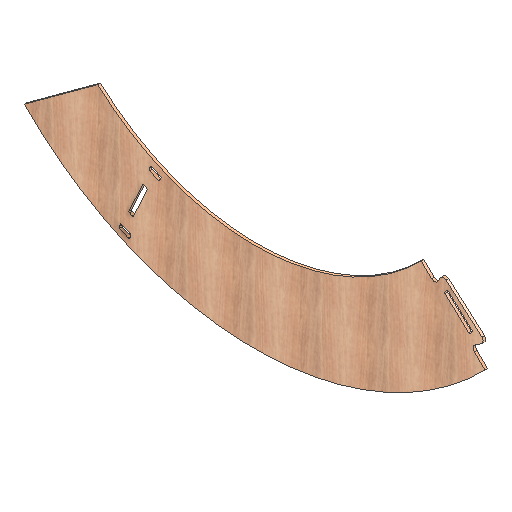
# Autodesk Inventor part: Platform C1
Saved by Autodesk Inventor 2021 (Build 250183000, 183)
## iProperties
Created: 2020-05-09
Part Number: Platform C1
Material: Wood (Birch)
Document SubType Name: Modeling
Designer: Dan Wikman
Density: 0.55 g/cm^3
Appearance: Birch - Natural Polished
Mass: 3085.21 g
Surface Area: 11708.7 cm^2
Volume: 5609.47 cm^3
Autodesk Inventor part; units mm, degrees
ref_plane "YZ Plane" through (0, 0, 0) normal (1, 0, 0) x (0, 1, 0)
ref_plane "XZ Plane" through (0, 0, 0) normal (0, 1, 0) x (-1, 0, 0)
ref_plane "XY Plane" through (0, 0, 0) normal (0, 0, 1) x (1, 0, 0)
sketch "CONTOURS" plane through (0, 0, 0) normal (0, 0, 1) x (1, 0, 0)
  line L0 (1957.6292, 879.0874) -> (1973.7702, 879.0874)
  arc A0 (1973.7702, 871.0874) -> (1973.7702, 879.0874) centre (1973.7702, 875.0874) ccw
  line L1 (2395.2631, 344.4855) -> (2395.2631, 361.2856)
  line L2 (2395.2631, 361.2856) -> (2335.4041, 361.2856)
  arc A1 (2327.4041, 361.2857) -> (2335.4041, 361.2856) centre (2331.4041, 361.2856) ccw
  line L3 (2327.4041, 361.2857) -> (2327.4041, 413.0854)
  arc A2 (2046.6196, 767.5507) -> (2327.4041, 413.0854) centre (2780.5524, 1060.4825) ccw
  arc A3 (2046.6196, 767.5507) -> (2038.9046, 766.0679) centre (2042.9046, 766.0679) ccw
  line L4 (2038.9046, 766.0679) -> (2038.9041, 604.8116)
  line L5 (2038.9041, 604.8116) -> (2060.9041, 604.8116)
  arc A4 (2068.9041, 604.8116) -> (2060.9041, 604.8116) centre (2064.9041, 604.8116) ccw
  line L6 (2068.9041, 604.8116) -> (2068.9041, 585.8116)
  arc A5 (2060.9041, 585.8116) -> (2068.9041, 585.8116) centre (2064.9041, 585.8116) ccw
  line L7 (2060.9041, 585.8116) -> (2037.4041, 585.8116)
  line L8 (2037.4041, 585.8116) -> (1996.4234, 585.8116)
  arc A6 (1988.9234, 587.8213) -> (1996.4234, 585.8116) centre (1996.4234, 600.8116) ccw
  line L9 (1988.9234, 587.8213) -> (1963.7631, 602.3475)
  arc A7 (1963.7631, 602.3475) -> (1957.7631, 598.8834) centre (1961.7631, 598.8834) ccw
  line L10 (1957.7631, 598.8834) -> (1957.7631, 403.7398)
  arc A8 (1957.7631, 403.7398) -> (1963.7631, 400.2757) centre (1961.7631, 403.7398) ccw
  line L11 (1963.7631, 400.2757) -> (1988.9234, 414.802)
  arc A9 (1996.4234, 416.8116) -> (1988.9234, 414.802) centre (1996.4234, 401.8116) ccw
  line L12 (1996.4234, 416.8116) -> (2037.4041, 416.8116)
  line L13 (2037.4041, 416.8116) -> (2060.9041, 416.8116)
  arc A10 (2068.9041, 416.8116) -> (2060.9041, 416.8116) centre (2064.9041, 416.8116) ccw
  line L14 (2068.9041, 416.8116) -> (2068.9041, 397.8116)
  arc A11 (2060.9041, 397.8116) -> (2068.9041, 397.8116) centre (2064.9041, 397.8116) ccw
  line L15 (2060.9041, 397.8116) -> (2038.9041, 397.8116)
  line L16 (2038.9041, 397.8116) -> (2038.9041, 210.8117)
  line L17 (2038.9041, 210.8117) -> (2052.4041, 210.8117)
  arc A12 (2052.4041, 202.8117) -> (2052.4041, 210.8117) centre (2052.4041, 206.8117) ccw
  line L18 (2052.4041, 202.8117) -> (2052.4041, 195.3488)
  arc A13 (2052.4041, 195.3488) -> (2327.4041, 47.9742) centre (2799.5688, 1259.2914) ccw
  arc A14 (2327.4041, 39.9742) -> (2327.4041, 47.9742) centre (2327.4041, 43.9742) ccw
  line L19 (2327.4041, 39.9742) -> (2327.4041, 23.2856)
  line L20 (2327.4041, 23.2856) -> (2395.2631, 23.2856)
  line L21 (2395.2631, 23.2856) -> (2395.2631, 40.0855)
  arc A15 (2395.2631, 48.0855) -> (2395.2631, 40.0855) centre (2395.2631, 44.0855) ccw
  line L22 (2395.2631, 48.0855) -> (2411.4041, 48.0855)
  line L23 (2411.4041, 48.0855) -> (2411.4041, 66.0855)
  line L24 (2411.4041, 66.0855) -> (2403.2631, 66.0855)
  arc A16 (2395.2631, 66.0855) -> (2403.2631, 66.0855) centre (2399.2631, 66.0855) ccw
  line L25 (2395.2631, 66.0855) -> (2395.2631, 132.0783)
  line L26 (2395.2631, 132.0783) -> (2373.2631, 132.0783)
  arc A17 (2365.2631, 132.0783) -> (2373.2631, 132.0783) centre (2369.2631, 132.0783) ccw
  line L27 (2365.2631, 132.0783) -> (2365.2631, 148.6501)
  line L28 (2365.2631, 148.6501) -> (2364.8394, 148.4335)
  line L29 (2364.8394, 148.4335) -> (2364.4234, 148.2026)
  line L30 (2364.4234, 148.2026) -> (2339.2631, 133.6763)
  arc A18 (2331.7631, 138.0065) -> (2339.2631, 133.6763) centre (2336.7631, 138.0065) ccw
  line L31 (2331.7631, 138.0065) -> (2331.7631, 246.5646)
  arc A19 (2339.2631, 250.8947) -> (2331.7631, 246.5646) centre (2336.7631, 246.5646) ccw
  line L32 (2339.2631, 250.8947) -> (2364.4234, 236.3684)
  line L33 (2364.4234, 236.3684) -> (2364.8394, 236.1375)
  line L34 (2364.8394, 236.1375) -> (2365.2631, 235.9209)
  line L35 (2365.2631, 235.9209) -> (2365.2631, 252.4928)
  arc A20 (2373.2631, 252.4928) -> (2365.2631, 252.4928) centre (2369.2631, 252.4928) ccw
  line L36 (2373.2631, 252.4928) -> (2395.2631, 252.4928)
  line L37 (2395.2631, 252.4928) -> (2395.2631, 318.4855)
  arc A21 (2403.2631, 318.4855) -> (2395.2631, 318.4855) centre (2399.2631, 318.4855) ccw
  line L38 (2403.2631, 318.4855) -> (2411.4041, 318.4855)
  line L39 (2411.4041, 318.4855) -> (2411.4041, 336.4855)
  line L40 (2411.4041, 336.4855) -> (2395.2631, 336.4855)
  arc A22 (2395.2631, 344.4855) -> (2395.2631, 336.4855) centre (2395.2631, 340.4855) ccw
  line L41 (1973.7702, 871.0874) -> (1973.7702, 854.2874)
  line L42 (1973.7702, 854.2874) -> (2033.6292, 854.2873)
  line L43 (2041.6292, 854.2873) -> (2041.6292, 802.4876)
  arc A23 (2322.4137, 448.0223) -> (2041.6292, 802.4876) centre (1588.4809, 155.0905) ccw
  arc A24 (2322.4137, 448.0223) -> (2330.1287, 449.505) centre (2326.1287, 449.505) ccw
  line L44 (2330.1287, 449.505) -> (2330.1292, 610.7613)
  line L45 (2330.1292, 610.7613) -> (2308.1292, 610.7613)
  arc A25 (2300.1292, 610.7613) -> (2308.1292, 610.7613) centre (2304.1292, 610.7613) ccw
  line L46 (2300.1292, 610.7613) -> (2300.1292, 629.7613)
  arc A26 (2308.1292, 629.7613) -> (2300.1292, 629.7613) centre (2304.1292, 629.7613) ccw
  line L47 (2308.1292, 629.7613) -> (2331.6292, 629.7613)
  line L48 (2331.6292, 629.7613) -> (2372.6099, 629.7613)
  arc A27 (2380.1099, 627.7517) -> (2372.6099, 629.7613) centre (2372.6099, 614.7613) ccw
  line L49 (2380.1099, 627.7517) -> (2405.2702, 613.2254)
  arc A28 (2405.2702, 613.2254) -> (2411.2702, 616.6895) centre (2407.2702, 616.6895) ccw
  line L50 (2411.2702, 616.6895) -> (2411.2702, 811.8331)
  line L51 (2405.2702, 815.2972) -> (2380.1099, 800.7709)
  arc A29 (2372.6099, 798.7613) -> (2380.1099, 800.7709) centre (2372.6099, 813.7613) ccw
  line L52 (2372.6099, 798.7613) -> (2331.6292, 798.7613)
  line L53 (2331.6292, 798.7613) -> (2308.1292, 798.7613)
  arc A30 (2300.1292, 798.7613) -> (2308.1292, 798.7613) centre (2304.1292, 798.7613) ccw
  line L54 (2300.1292, 798.7613) -> (2300.1292, 817.7613)
  arc A31 (2308.1292, 817.7613) -> (2300.1292, 817.7613) centre (2304.1292, 817.7613) ccw
  line L55 (2308.1292, 817.7613) -> (2330.1292, 817.7613)
  line L56 (2330.1292, 817.7613) -> (2330.1292, 1004.7612)
  line L57 (2330.1292, 1004.7612) -> (2316.6292, 1004.7612)
  arc A32 (2316.6292, 1012.7612) -> (2316.6292, 1004.7612) centre (2316.6292, 1008.7612) ccw
  line L58 (2316.6292, 1012.7612) -> (2316.6292, 1020.2242)
  arc A33 (2316.6292, 1020.2242) -> (2041.6292, 1167.5988) centre (1569.4645, -43.7184) ccw
  arc A34 (2041.6292, 1175.5988) -> (2041.6292, 1167.5988) centre (2041.6292, 1171.5988) ccw
  line L59 (2041.6292, 1175.5988) -> (2041.6292, 1192.2873)
  line L60 (2041.6292, 1192.2873) -> (1973.7702, 1192.2873)
  line L61 (1973.7702, 1192.2873) -> (1973.7702, 1175.4874)
  arc A35 (1973.7702, 1167.4874) -> (1973.7702, 1175.4874) centre (1973.7702, 1171.4874) ccw
  line L62 (1973.7702, 1167.4874) -> (1957.6292, 1167.4874)
  line L63 (1957.6292, 1167.4874) -> (1957.6292, 1149.4874)
  line L64 (1957.6292, 1149.4874) -> (1965.7702, 1149.4874)
  arc A36 (1973.7702, 1149.4874) -> (1965.7702, 1149.4874) centre (1969.7702, 1149.4874) ccw
  line L65 (1973.7702, 1149.4874) -> (1973.7702, 1083.4947)
  line L66 (1973.7702, 1083.4947) -> (1995.7702, 1083.4947)
  arc A37 (2003.7702, 1083.4946) -> (1995.7702, 1083.4947) centre (1999.7702, 1083.4947) ccw
  line L67 (2003.7702, 1083.4946) -> (2003.7702, 1066.9228)
  line L68 (2003.7702, 1066.9228) -> (2004.1939, 1067.1394)
  line L69 (2004.1939, 1067.1394) -> (2004.6099, 1067.3703)
  line L70 (2004.6099, 1067.3703) -> (2029.7702, 1081.8966)
  arc A38 (2037.2702, 1077.5665) -> (2029.7702, 1081.8966) centre (2032.2702, 1077.5665) ccw
  line L71 (2037.2702, 1077.5665) -> (2037.2702, 969.0084)
  line L72 (2029.7702, 964.6782) -> (2004.6099, 979.2045)
  line L73 (2004.6099, 979.2045) -> (2004.1939, 979.4354)
  line L74 (2004.1939, 979.4354) -> (2003.7702, 979.652)
  line L75 (2003.7702, 979.652) -> (2003.7702, 963.0802)
  arc A39 (1995.7702, 963.0802) -> (2003.7702, 963.0802) centre (1999.7702, 963.0802) ccw
  arc A40 (2411.2702, 811.8331) -> (2405.2702, 815.2972) centre (2407.2702, 811.8331) ccw
  line L76 (29.0412, 889.8609) -> (69.6135, 929.6413)
  arc A41 (92.1865, 926.768) -> (69.6135, 929.6413) centre (79.765, 919.2877) ccw
  line L77 (92.1865, 926.768) -> (107.0781, 902.0398)
  arc A42 (107.0781, 902.0398) -> (131.8211, 899.605) centre (120.3563, 910.0361) ccw
  line L78 (131.8211, 899.605) -> (252.9238, 1032.7101)
  arc A43 (252.9238, 1032.7101) -> (248.9601, 1056.7052) centre (241.459, 1043.1412) ccw
  line L79 (248.9601, 1056.7052) -> (234.1791, 1064.8793)
  arc A44 (231.0447, 1087.9218) -> (234.1791, 1064.8793) centre (241.1963, 1077.5683) ccw
  line L80 (231.0447, 1087.9218) -> (270.3869, 1126.4961)
  arc A45 (270.3869, 1126.4961) -> (1527.2637, 1126.4961) centre (898.8253, 1743.5906) ccw
  line L81 (1527.2637, 1126.4961) -> (1815.1018, 939.9773)
  arc A46 (29.0412, 889.8609) -> (1815.1018, 939.9773) centre (898.8169, 1743.6721) ccw
  line L82 (1523.2972, 649.9931) -> (1562.6322, 611.4115)
  arc A47 (1562.6322, 611.4115) -> (1587.1937, 615.2422) centre (1573.4858, 622.4771) ccw
  line L83 (1587.1937, 615.2422) -> (1595.0777, 630.18)
  arc A48 (1617.4481, 634.3255) -> (1595.0777, 630.18) centre (1607.9012, 623.4119) ccw
  line L84 (1617.4481, 634.3255) -> (1752.8919, 515.8444)
  arc A49 (1751.0665, 492.6576) -> (1752.8919, 515.8444) centre (1743.3451, 504.9307) ccw
  line L85 (1751.0665, 492.6576) -> (1726.6337, 477.2861)
  arc A50 (1726.6337, 477.2861) -> (1724.034, 453.1009) centre (1734.8877, 464.1665) ccw
  line L86 (1724.034, 453.1009) -> (1764.599, 413.3129)
  arc A51 (25.3482, 413.3129) -> (1764.599, 413.3129) centre (894.9736, 1267.2896) ccw
  line L87 (25.3482, 413.3129) -> (302.205, 615.759)
  arc A52 (302.205, 615.759) -> (1523.2972, 649.9931) centre (894.9664, 1267.2343) ccw
  line L88 (1995.7702, 963.0802) -> (1973.7702, 963.0802)
  line L89 (1973.7702, 963.0802) -> (1973.7702, 897.0874)
  arc A53 (1965.7702, 897.0874) -> (1973.7702, 897.0874) centre (1969.7702, 897.0874) ccw
  line L90 (1965.7702, 897.0874) -> (1957.6292, 897.0874)
  line L91 (1957.6292, 897.0874) -> (1957.6292, 879.0874)
  dimension "d1" = 338
  dimension "d3" = 16.6885
  dimension "d5" = 18
  dimension "d7" = 16.141
  dimension "d9" = 51.7997
  dimension "d11" = 1300.088
  dimension "d13" = 16.7999
  constraints: 184 end point, 108 point on circle, 54 centre point
  measures "d1" distance of L43.start L59.end
  measures "d3" distance of L59.start L59.end
  measures "d5" distance of L90.end L0.start
  measures "d7" distance from line of L89 L90.end
  measures "d9" distance of L43.start L43.end
  measures "d11" radius of A33
  measures "d13" distance of L60.end L61.end
sketch "HOLES" plane through (0, 0, 0) normal (0, 0, 1) x (1, 0, 0)
  line L0 (417.6052, 171.9081) -> (384.9317, 187.0224)
  arc A0 (382.9807, 192.3322) -> (384.9317, 187.0224) centre (386.6111, 190.6528) ccw
  line L1 (382.9807, 192.3322) -> (387.5989, 202.3157)
  arc A1 (392.9087, 204.2668) -> (387.5989, 202.3157) centre (391.2293, 200.6364) ccw
  line L2 (392.9087, 204.2668) -> (425.5822, 189.1525)
  arc A2 (427.5332, 183.8427) -> (425.5822, 189.1525) centre (423.9028, 185.5221) ccw
  line L3 (290.0252, 1067.7256) -> (282.3828, 1059.8139)
  arc A3 (276.7268, 1059.716) -> (282.3828, 1059.8139) centre (279.5059, 1062.593) ccw
  line L4 (276.7268, 1059.716) -> (250.8342, 1084.7274)
  arc A4 (250.7363, 1090.3834) -> (250.8342, 1084.7274) centre (253.6132, 1087.6044) ccw
  line L5 (250.7363, 1090.3834) -> (258.3786, 1098.2951)
  arc A5 (264.0347, 1098.393) -> (258.3786, 1098.2951) centre (261.2556, 1095.516) ccw
  line L6 (264.0347, 1098.393) -> (289.9273, 1073.3816)
  arc A6 (290.0252, 1067.7256) -> (289.9273, 1073.3816) centre (287.1482, 1070.5046) ccw
  line L7 (102.1615, 873.2431) -> (94.5191, 865.3315)
  arc A7 (88.8631, 865.2335) -> (94.5191, 865.3315) centre (91.6422, 868.1105) ccw
  line L8 (88.8631, 865.2335) -> (62.9705, 890.245)
  arc A8 (62.8726, 895.901) -> (62.9705, 890.245) centre (65.7496, 893.1219) ccw
  line L9 (62.8726, 895.901) -> (70.515, 903.8126)
  arc A9 (76.171, 903.9105) -> (70.515, 903.8126) centre (73.3919, 901.0336) ccw
  line L10 (488.8536, 364.5631) -> (437.7587, 253.7781)
  arc A10 (102.1615, 873.2431) -> (102.0636, 878.8991) centre (99.2846, 876.0221) ccw
  line L11 (1358.4331, 945.869) -> (1353.2703, 955.5821)
  arc A11 (1353.2703, 955.5821) -> (1347.8609, 957.2368) centre (1349.7382, 953.7047) ccw
  line L12 (1347.8609, 957.2368) -> (1316.0723, 940.3404)
  arc A12 (1316.0723, 940.3404) -> (1314.4176, 934.931) centre (1317.9497, 936.8084) ccw
  line L13 (1314.4176, 934.931) -> (1319.5804, 925.2178)
  arc A13 (1319.5804, 925.2178) -> (1324.9899, 923.5631) centre (1323.1125, 927.0952) ccw
  line L14 (1324.9899, 923.5631) -> (1356.7784, 940.4595)
  arc A14 (1356.7784, 940.4595) -> (1358.4331, 945.869) centre (1354.901, 943.9916) ccw
  line L15 (1441.3284, 696.1636) -> (1446.4912, 686.4505)
  arc A15 (1446.4912, 686.4505) -> (1451.9006, 684.7958) centre (1450.0232, 688.3278) ccw
  line L16 (1451.9006, 684.7958) -> (1483.6892, 701.6922)
  arc A16 (1483.6892, 701.6922) -> (1485.3438, 707.1016) centre (1481.8118, 705.2242) ccw
  line L17 (1485.3438, 707.1016) -> (1480.181, 716.8148)
  arc A17 (1480.181, 716.8148) -> (1474.7716, 718.4695) centre (1476.649, 714.9374) ccw
  line L18 (1474.7716, 718.4695) -> (1442.9831, 701.5731)
  arc A18 (1442.9831, 701.5731) -> (1441.3284, 696.1636) centre (1444.8604, 698.041) ccw
  line L19 (1363.2554, 875.1779) -> (1357.078, 871.8854)
  arc A19 (1357.078, 871.8854) -> (1355.4295, 866.4741) centre (1358.9594, 868.3555) ccw
  line L20 (1355.4295, 866.4741) -> (1412.8118, 758.8114)
  arc A20 (1412.8118, 758.8114) -> (1418.2231, 757.1628) centre (1416.3417, 760.6927) ccw
  line L21 (1418.2231, 757.1628) -> (1427.9304, 762.3366)
  arc A21 (1427.9304, 762.3366) -> (1429.579, 767.7479) centre (1426.049, 765.8666) ccw
  line L22 (1429.579, 767.7479) -> (1372.1967, 875.4107)
  arc A22 (1372.1967, 875.4107) -> (1366.7853, 877.0592) centre (1368.6667, 873.5293) ccw
  line L23 (1366.7853, 877.0592) -> (1363.2554, 875.1779)
  line L24 (1703.0768, 505.0739) -> (1613.5973, 588.0042)
  arc A23 (1613.3826, 593.657) -> (1613.5973, 588.0042) centre (1616.3164, 590.938) ccw
  line L25 (1613.3826, 593.657) -> (1620.8599, 601.7248)
  arc A24 (1626.5127, 601.9395) -> (1620.8599, 601.7248) centre (1623.7937, 599.0058) ccw
  line L26 (1626.5127, 601.9395) -> (1715.9922, 519.0093)
  arc A25 (1716.2069, 513.3565) -> (1715.9922, 519.0093) centre (1713.2731, 516.0755) ccw
  line L27 (1716.2069, 513.3565) -> (1708.7296, 505.2887)
  arc A26 (1703.0768, 505.0739) -> (1708.7296, 505.2887) centre (1705.7958, 508.0077) ccw
  line L28 (541.1297, 429.4206) -> (541.1463, 429.4626)
  arc A27 (541.1463, 429.4626) -> (539.1072, 434.5669) centre (537.4278, 430.9365) ccw
  line L29 (539.1072, 434.5669) -> (506.4339, 449.6811)
  arc A28 (506.4339, 449.6811) -> (501.1241, 447.7301) centre (504.7545, 446.0507) ccw
  line L30 (501.1241, 447.7301) -> (496.5059, 437.7465)
  arc A29 (496.5059, 437.7465) -> (498.4569, 432.4368) centre (500.1363, 436.0672) ccw
  line L31 (498.4569, 432.4368) -> (531.1304, 417.3225)
  arc A30 (531.1304, 417.3225) -> (536.4402, 419.2735) centre (532.8098, 420.9529) ccw
  line L32 (536.4402, 419.2735) -> (541.0584, 429.2571)
  line L33 (541.0584, 429.2571) -> (541.0948, 429.338)
  line L34 (541.0948, 429.338) -> (541.1297, 429.4206)
  line L35 (480.54, 372.8023) -> (486.8965, 369.8706)
  arc A31 (488.8536, 364.5631) -> (486.8965, 369.8706) centre (485.2213, 366.2383) ccw
  arc A32 (432.4511, 251.8211) -> (437.7587, 253.7781) centre (434.1264, 255.4533) ccw
  line L36 (432.4511, 251.8211) -> (422.4623, 256.428)
  arc A33 (420.5053, 261.7355) -> (422.4623, 256.428) centre (424.1376, 260.0603) ccw
  line L37 (420.5053, 261.7355) -> (471.6002, 372.5205)
  arc A34 (476.9077, 374.4775) -> (471.6002, 372.5205) centre (475.2325, 370.8452) ccw
  line L38 (476.9077, 374.4775) -> (480.54, 372.8023)
  line L39 (427.5332, 183.8427) -> (422.915, 173.8591)
  arc A35 (417.6052, 171.9081) -> (422.915, 173.8591) centre (419.2846, 175.5385) ccw
  line L40 (76.171, 903.9105) -> (102.0636, 878.8991)
  constraints: 82 end point, 72 point on circle, 36 centre point
sketch "LETTERS" plane through (0, 0, 0) normal (0, 0, 1) x (1, 0, 0)
  line L0 (565.2488, 269.5965) -> (565.4715, 269.5068)
  line L1 (565.4715, 269.5068) -> (565.6923, 269.4126)
  line L2 (565.6923, 269.4126) -> (565.9113, 269.314)
  line L3 (565.9113, 269.314) -> (566.1283, 269.2109)
  line L4 (566.1283, 269.2109) -> (566.3432, 269.1036)
  line L5 (566.3432, 269.1036) -> (566.556, 268.9919)
  line L6 (566.556, 268.9919) -> (566.7665, 268.876)
  line L7 (566.7665, 268.876) -> (566.9747, 268.7559)
  line L8 (566.9747, 268.7559) -> (567.1804, 268.6317)
  line L9 (567.1804, 268.6317) -> (567.3837, 268.5035)
  line L10 (567.3837, 268.5035) -> (567.5843, 268.3713)
  line L11 (567.5843, 268.3713) -> (567.7822, 268.2351)
  line L12 (567.7822, 268.2351) -> (567.9773, 268.095)
  line L13 (567.9773, 268.095) -> (568.1695, 267.951)
  line L14 (568.1695, 267.951) -> (568.3587, 267.8033)
  line L15 (568.3587, 267.8033) -> (568.5449, 267.6519)
  line L16 (568.5449, 267.6519) -> (568.7279, 267.4968)
  line L17 (568.7279, 267.4968) -> (568.9076, 267.3381)
  line L18 (568.9076, 267.3381) -> (569.084, 267.1758)
  line L19 (569.084, 267.1758) -> (569.2569, 267.01)
  line L20 (569.2569, 267.01) -> (569.4263, 266.8407)
  line L21 (569.4263, 266.8407) -> (569.5921, 266.6681)
  line L22 (569.5921, 266.6681) -> (569.7542, 266.4921)
  line L23 (569.7542, 266.4921) -> (569.9124, 266.3129)
  line L24 (569.9124, 266.3129) -> (570.0668, 266.1304)
  line L25 (570.0668, 266.1304) -> (570.2171, 265.9448)
  line L26 (570.2171, 265.9448) -> (570.3634, 265.756)
  line L27 (570.3634, 265.756) -> (570.5054, 265.5642)
  line L28 (570.5054, 265.5642) -> (570.6432, 265.3693)
  line L29 (570.6432, 265.3693) -> (570.7767, 265.1716)
  line L30 (570.7767, 265.1716) -> (570.9058, 264.9711)
  line L31 (570.9058, 264.9711) -> (571.0303, 264.7679)
  line L32 (571.0303, 264.7679) -> (571.1503, 264.5622)
  line L33 (571.1503, 264.5622) -> (571.2656, 264.354)
  line L34 (571.2656, 264.354) -> (571.3762, 264.1435)
  line L35 (571.3762, 264.1435) -> (571.482, 263.9307)
  line L36 (571.482, 263.9307) -> (571.583, 263.7158)
  line L37 (571.583, 263.7158) -> (571.679, 263.4989)
  line L38 (571.679, 263.4989) -> (571.77, 263.28)
  line L39 (571.77, 263.28) -> (571.8558, 263.0594)
  line L40 (571.8558, 263.0594) -> (571.9365, 262.8371)
  line L41 (571.9365, 262.8371) -> (572.012, 262.6132)
  line L42 (572.012, 262.6132) -> (572.0821, 262.3878)
  line L43 (572.0821, 262.3878) -> (572.1469, 262.1611)
  line L44 (572.1469, 262.1611) -> (572.2061, 261.9332)
  line L45 (572.2061, 261.9332) -> (572.2599, 261.7041)
  line L46 (572.2599, 261.7041) -> (572.308, 261.474)
  line L47 (572.308, 261.474) -> (572.3504, 261.2429)
  line L48 (572.3504, 261.2429) -> (572.3871, 261.0111)
  line L49 (572.3871, 261.0111) -> (572.4179, 260.7785)
  line L50 (572.4179, 260.7785) -> (572.4428, 260.5454)
  line L51 (572.4428, 260.5454) -> (572.4617, 260.3118)
  line L52 (572.4617, 260.3118) -> (572.4745, 260.0778)
  line L53 (572.4745, 260.0778) -> (572.4811, 259.8435)
  line L54 (572.4811, 259.8435) -> (572.4816, 259.6092)
  line L55 (572.4816, 259.6092) -> (572.4757, 259.3747)
  line L56 (572.4757, 259.3747) -> (572.4635, 259.1404)
  line L57 (572.4635, 259.1404) -> (572.4449, 258.9062)
  line L58 (572.4449, 258.9062) -> (572.4197, 258.6723)
  line L59 (572.4197, 258.6723) -> (572.3879, 258.4388)
  line L60 (572.3879, 258.4388) -> (572.3494, 258.2058)
  line L61 (572.3494, 258.2058) -> (572.3044, 257.9735)
  line L62 (572.3044, 257.9735) -> (572.2529, 257.7421)
  line L63 (572.2529, 257.7421) -> (572.195, 257.5116)
  line L64 (572.195, 257.5116) -> (572.1308, 257.2824)
  line L65 (572.1308, 257.2824) -> (572.0604, 257.0546)
  line L66 (572.0604, 257.0546) -> (571.9839, 256.8283)
  line L67 (571.9839, 256.8283) -> (571.9014, 256.6037)
  line L68 (571.9014, 256.6037) -> (571.8129, 256.381)
  line L69 (571.8129, 256.381) -> (571.7186, 256.1604)
  line L70 (571.7186, 256.1604) -> (571.6186, 255.9421)
  line L71 (571.6186, 255.9421) -> (571.5129, 255.7261)
  line L72 (571.5129, 255.7261) -> (571.4016, 255.5127)
  line L73 (571.4016, 255.5127) -> (571.2849, 255.3021)
  line L74 (571.2849, 255.3021) -> (571.1628, 255.0944)
  line L75 (571.1628, 255.0944) -> (571.0354, 254.8898)
  line L76 (571.0354, 254.8898) -> (570.9028, 254.6885)
  line L77 (570.9028, 254.6885) -> (570.7652, 254.4906)
  line L78 (570.7652, 254.4906) -> (570.6225, 254.2964)
  line L79 (570.6225, 254.2964) -> (570.4749, 254.106)
  line L80 (570.4749, 254.106) -> (570.3225, 253.9195)
  line L81 (570.3225, 253.9195) -> (570.1654, 253.7372)
  line L82 (570.1654, 253.7372) -> (570.0037, 253.5591)
  line L83 (570.0037, 253.5591) -> (569.8374, 253.3856)
  line L84 (569.8374, 253.3856) -> (569.6667, 253.2167)
  line L85 (569.6667, 253.2167) -> (569.4916, 253.0527)
  line L86 (569.4916, 253.0527) -> (569.3123, 252.8937)
  line L87 (569.3123, 252.8937) -> (569.1288, 252.7398)
  line L88 (569.1288, 252.7398) -> (568.9412, 252.5913)
  line L89 (568.9412, 252.5913) -> (568.7497, 252.4483)
  line L90 (568.7497, 252.4483) -> (568.5543, 252.311)
  line L91 (568.5543, 252.311) -> (568.355, 252.1796)
  line L92 (568.355, 252.1796) -> (568.1521, 252.0542)
  line L93 (568.1521, 252.0542) -> (567.9457, 251.9349)
  line L94 (567.9457, 251.9349) -> (567.736, 251.8219)
  line L95 (567.736, 251.8219) -> (567.5231, 251.715)
  line L96 (567.5231, 251.715) -> (567.3073, 251.6145)
  line L97 (567.3073, 251.6145) -> (567.0888, 251.5204)
  line L98 (567.0888, 251.5204) -> (566.8677, 251.4327)
  line L99 (566.8677, 251.4327) -> (566.6443, 251.3516)
  line L100 (566.6443, 251.3516) -> (566.4187, 251.2771)
  line L101 (566.4187, 251.2771) -> (566.1911, 251.2092)
  line L102 (566.1911, 251.2092) -> (565.9618, 251.1481)
  line L103 (565.9618, 251.1481) -> (565.7308, 251.0938)
  line L104 (565.7308, 251.0938) -> (565.4985, 251.0464)
  line L105 (565.4985, 251.0464) -> (565.265, 251.0059)
  line L106 (565.265, 251.0059) -> (565.0305, 250.9724)
  line L107 (565.0305, 250.9724) -> (564.7951, 250.946)
  line L108 (564.7951, 250.946) -> (564.5591, 250.9268)
  line L109 (564.5591, 250.9268) -> (564.3227, 250.9148)
  line L110 (564.3227, 250.9148) -> (564.0861, 250.9101)
  line L111 (564.0861, 250.9101) -> (563.8494, 250.9127)
  line L112 (563.8494, 250.9127) -> (563.6128, 250.9228)
  line L113 (563.6128, 250.9228) -> (563.3766, 250.9404)
  line L114 (563.1409, 250.9656) -> (562.906, 250.9983)
  line L115 (562.906, 250.9983) -> (562.6719, 251.0388)
  line L116 (562.6719, 251.0388) -> (562.439, 251.0871)
  line L117 (562.439, 251.0871) -> (562.2074, 251.1432)
  line L118 (562.2074, 251.1432) -> (561.9772, 251.2072)
  line L119 (561.9772, 251.2072) -> (561.7487, 251.2792)
  line L120 (561.7487, 251.2792) -> (561.5221, 251.3592)
  line L121 (561.5221, 251.3592) -> (561.2975, 251.4473)
  line L122 (561.2975, 251.4473) -> (561.1861, 251.4945)
  line L123 (561.1861, 251.4945) -> (561.0753, 251.5437)
  line L124 (554.4697, 256.2412) -> (554.3188, 256.4266)
  line L125 (554.3188, 256.4266) -> (554.1731, 256.616)
  line L126 (554.1731, 256.616) -> (554.0329, 256.8093)
  line L127 (554.0329, 256.8093) -> (553.898, 257.0063)
  line L128 (553.898, 257.0063) -> (553.7686, 257.2069)
  line L129 (553.7686, 257.2069) -> (553.6447, 257.411)
  line L130 (553.6447, 257.411) -> (553.5265, 257.6182)
  line L131 (553.5265, 257.6182) -> (553.414, 257.8286)
  line L132 (553.414, 257.8286) -> (553.3071, 258.0418)
  line L133 (553.3071, 258.0418) -> (553.2061, 258.2578)
  line L134 (553.2061, 258.2578) -> (553.1109, 258.4764)
  line L135 (553.1109, 258.4764) -> (553.0217, 258.6974)
  line L136 (553.0217, 258.6974) -> (552.9385, 258.9206)
  line L137 (552.9385, 258.9206) -> (552.8613, 259.1459)
  line L138 (552.8613, 259.1459) -> (552.7902, 259.3732)
  line L139 (563.3766, 250.9404) -> (563.1409, 250.9656)
  line L140 (552.7902, 259.3732) -> (552.7253, 259.6021)
  line L141 (552.7253, 259.6021) -> (552.6667, 259.8327)
  line L142 (552.6667, 259.8327) -> (552.6143, 260.0646)
  line L143 (552.6143, 260.0646) -> (552.5684, 260.2978)
  line L144 (552.5684, 260.2978) -> (552.5289, 260.5321)
  line L145 (552.5289, 260.5321) -> (552.4959, 260.7673)
  line L146 (552.4959, 260.7673) -> (552.4694, 261.0032)
  line L147 (552.4694, 261.0032) -> (552.4496, 261.2397)
  line L148 (552.4496, 261.2397) -> (552.4365, 261.4766)
  line L149 (552.4365, 261.4766) -> (552.4301, 261.7138)
  line L150 (552.4301, 261.7138) -> (552.4305, 261.9511)
  line L151 (552.4305, 261.9511) -> (552.4379, 262.1882)
  line L152 (552.4379, 262.1882) -> (552.4522, 262.4251)
  line L153 (552.4522, 262.4251) -> (552.4735, 262.6616)
  line L154 (552.4735, 262.6616) -> (552.5018, 262.8975)
  line L155 (552.5018, 262.8975) -> (552.5373, 263.1327)
  line L156 (552.5373, 263.1327) -> (552.5801, 263.3669)
  line L157 (552.5801, 263.3669) -> (552.63, 263.6001)
  line L158 (552.63, 263.6001) -> (552.6871, 263.832)
  line L159 (552.6871, 263.832) -> (552.7512, 264.0625)
  line L160 (552.7512, 264.0625) -> (552.8221, 264.2913)
  line L161 (552.8221, 264.2913) -> (552.8997, 264.5184)
  line L162 (552.8997, 264.5184) -> (552.9838, 264.7436)
  line L163 (552.9838, 264.7436) -> (553.0744, 264.9667)
  line L164 (553.0744, 264.9667) -> (553.1713, 265.1875)
  line L165 (553.1713, 265.1875) -> (553.2743, 265.4059)
  line L166 (553.2743, 265.4059) -> (553.3833, 265.6216)
  line L167 (553.3833, 265.6216) -> (553.4982, 265.8346)
  line L168 (553.4982, 265.8346) -> (553.6188, 266.0446)
  line L169 (553.6188, 266.0446) -> (553.745, 266.2515)
  line L170 (553.745, 266.2515) -> (553.8766, 266.4551)
  line L171 (553.8766, 266.4551) -> (554.0134, 266.6552)
  line L172 (554.0134, 266.6552) -> (554.1555, 266.8517)
  line L173 (554.1555, 266.8517) -> (554.3025, 267.0444)
  line L174 (554.3025, 267.0444) -> (554.4545, 267.2331)
  line L175 (554.4545, 267.2331) -> (554.6111, 267.4177)
  line L176 (554.6111, 267.4177) -> (554.7724, 267.598)
  line L177 (554.7724, 267.598) -> (554.9381, 267.7738)
  line L178 (554.9381, 267.7738) -> (555.108, 267.945)
  line L179 (555.108, 267.945) -> (555.2822, 268.1113)
  line L180 (555.2822, 268.1113) -> (555.4604, 268.2726)
  line L181 (555.4604, 268.2726) -> (555.6425, 268.4288)
  line L182 (555.6425, 268.4288) -> (555.8283, 268.5797)
  line L183 (555.8283, 268.5797) -> (556.0177, 268.725)
  line L184 (556.0177, 268.725) -> (556.2106, 268.8647)
  line L185 (556.2106, 268.8647) -> (556.4068, 268.9986)
  line L186 (556.4068, 268.9986) -> (556.6061, 269.1264)
  line L187 (556.6061, 269.1264) -> (556.8085, 269.2481)
  line L188 (556.8085, 269.2481) -> (557.0138, 269.3634)
  line L189 (557.0138, 269.3634) -> (557.2219, 269.4722)
  line L190 (557.2219, 269.4722) -> (557.4326, 269.5746)
  line L191 (557.4326, 269.5746) -> (557.6458, 269.6706)
  line L192 (557.6458, 269.6706) -> (557.8613, 269.7602)
  line L193 (557.8613, 269.7602) -> (558.0792, 269.8435)
  line L194 (558.0792, 269.8435) -> (558.2991, 269.9206)
  line L195 (558.2991, 269.9206) -> (558.521, 269.9914)
  line L196 (558.521, 269.9914) -> (558.7448, 270.0562)
  line L197 (558.7448, 270.0562) -> (558.9703, 270.1148)
  line L198 (558.9703, 270.1148) -> (559.1974, 270.1675)
  line L199 (559.1974, 270.1675) -> (559.426, 270.2141)
  line L200 (559.426, 270.2141) -> (559.6559, 270.2548)
  line L201 (559.6559, 270.2548) -> (559.8871, 270.2897)
  line L202 (559.8871, 270.2897) -> (560.1194, 270.3188)
  line L203 (560.1194, 270.3188) -> (560.3526, 270.342)
  line L204 (560.3526, 270.342) -> (560.5867, 270.3596)
  line L205 (560.5867, 270.3596) -> (560.8215, 270.3716)
  line L206 (560.8215, 270.3716) -> (561.0569, 270.3779)
  line L207 (561.0569, 270.3779) -> (561.2927, 270.3787)
  line L208 (561.2927, 270.3787) -> (561.5289, 270.374)
  line L209 (561.5289, 270.374) -> (561.7653, 270.3638)
  line L210 (561.7653, 270.3638) -> (562.0017, 270.3483)
  line L211 (562.0017, 270.3483) -> (562.2381, 270.3274)
  line L212 (562.2381, 270.3274) -> (562.4743, 270.3013)
  line L213 (562.4743, 270.3013) -> (562.7102, 270.27)
  line L214 (562.7102, 270.27) -> (562.9457, 270.2335)
  line L215 (562.9457, 270.2335) -> (563.1806, 270.1919)
  line L216 (563.1806, 270.1919) -> (563.4148, 270.1452)
  line L217 (563.4148, 270.1452) -> (563.6483, 270.0936)
  line L218 (563.6483, 270.0936) -> (563.8807, 270.037)
  line L219 (563.8807, 270.037) -> (564.1121, 269.9755)
  line L220 (564.1121, 269.9755) -> (564.3423, 269.9091)
  line L221 (564.3423, 269.9091) -> (564.5711, 269.838)
  line L222 (564.5711, 269.838) -> (564.7986, 269.7622)
  line L223 (564.7986, 269.7622) -> (565.0245, 269.6817)
  line L224 (565.0245, 269.6817) -> (565.2488, 269.5965)
  constraints: 450 end point, 5 perpendicular
extrude "Extrusion1" add sketch "CONTOURS" along normal blind 10 contours L82 A47 L83 A48 L84 A49 L85 A50 L86 A51 L87 A52
extrude "Extrusion2" cut sketch "HOLES" along normal blind 18 contours L0 A0 L1 A1 L2 A2 L39 A35 | L10 A32 L36 A33 L37 A34 L38 L35 A31 | L24 A23 L25 A24 L26 A25 L27 A26 | L34 L33 L32 A30 L31 A29 L30 A28 L29 A27 L28
body "Solid1"
